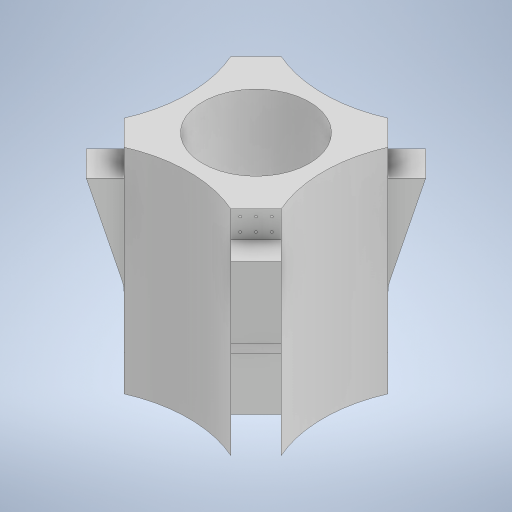
# Autodesk Inventor part: Table Base X1
Saved by Autodesk Inventor 2023 (Build 270158000, 158)
## iProperties
Created: 2022-11-22
Part Number: Table Base X1
Material: Generic
Document SubType Name: Modeling
Designer: surat
Density: 1 g/cm^3
Appearance: Default
Author: surat
Autodesk Inventor part; units mm, degrees
ref_plane "YZ Plane" through (0, 0, 0) normal (1, 0, 0) x (0, 1, 0)
ref_plane "XZ Plane" through (0, 0, 0) normal (0, 1, 0) x (-1, 0, 0)
sketch "Sketch1" plane through (0, 0, 0) normal (0, 1, 0) x (-1, 0, 0)
  line L0 (6.35, 0) -> (1365.25, 0)
  line L1 (1371.6, -6.35) -> (1371.6, -1365.25)
  line L2 (1365.25, -1371.6) -> (6.35, -1371.6)
  line L3 (0, -1365.25) -> (0, -6.35)
  line L4 (1346.2, -1346.2) -> (1346.2, -25.4)
  line L5 (1346.2, -25.4) -> (25.4, -25.4)
  line L6 (25.4, -25.4) -> (25.4, -1346.2)
  line L7 (25.4, -1346.2) -> (1346.2, -1346.2)
  line L8 (1320.8, -50.8) -> (1320.8, -1320.8)
  line L9 (1320.8, -1320.8) -> (50.8, -1320.8)
  line L10 (50.8, -1320.8) -> (50.8, -50.8)
  line L11 (50.8, -50.8) -> (1320.8, -50.8)
  line L12 (1320.8, -50.8) -> (1346.2, -25.4)
  line L13 (1320.8, -1320.8) -> (1346.2, -1346.2)
  line L14 (50.8, -1320.8) -> (25.4, -1346.2)
  line L15 (50.8, -50.8) -> (25.4, -25.4)
  line L16 (1365.25, 0) -> (1371.6, -6.35)
  line L17 (1371.6, -1365.25) -> (1365.25, -1371.6)
  line L18 (6.35, -1371.6) -> (0, -1365.25)
  line L19 (6.35, 0) -> (0, -6.35)
  line L20 (1320.8, -50.8) -> (50.8, -1320.8)
  line L21 (1320.8, -1320.8) -> (50.8, -50.8)
  line L22 (1320.8, -122.642049) -> (122.642049, -1320.8)
  line L23 (50.8, -1248.957951) -> (1248.957951, -50.8)
  line L24 (50.8, -122.642049) -> (1248.957951, -1320.8)
  line L25 (1320.8, -1248.957951) -> (122.642049, -50.8)
  line L26 (910.042049, -533.4) -> (910.042049, -838.2)
  line L27 (838.2, -910.042049) -> (533.4, -910.042049)
  line L28 (461.557951, -838.2) -> (461.557951, -533.4)
  line L29 (838.2, -461.557951) -> (533.4, -461.557951)
  line L30 (838.2, -461.557951) -> (910.042049, -533.4)
  line L31 (910.042049, -838.2) -> (838.2, -910.042049)
  line L32 (533.4, -910.042049) -> (461.557951, -838.2)
  line L33 (461.557951, -533.4) -> (533.4, -461.557951)
  arc A0 (910.042049, -533.4) -> (910.042049, -838.2) centre (1259.234317, -685.8) ccw
  arc A1 (838.2, -910.042049) -> (533.4, -910.042049) centre (685.8, -1259.234317) ccw
  arc A2 (461.557951, -838.2) -> (461.557951, -533.4) centre (112.365683, -685.8) ccw
  arc A3 (533.4, -461.557951) -> (838.2, -461.557951) centre (685.8, -112.365683) ccw
  point P0 (0, 0)
  point P1 (1371.6, -1371.6)
  point P2 (1371.6, 0)
  point P3 (0, -1371.6)
  dimension "d0" = 1371.6
  dimension "d1" = 1371.6
  dimension "d2" = 25.4
  dimension "d3" = 25.4
  dimension "d34" = 6.35
  dimension "d35" = 6.35
  dimension "d36" = 6.35
  dimension "d37" = 6.35
  dimension "d38" = 6.35
  dimension "d39" = 6.35
  dimension "d40" = 6.35
  dimension "d41" = 6.35
  dimension "d42" = 50.8
  dimension "d43" = 50.8
  dimension "d44" = 50.8
  dimension "d45" = 50.8
  dimension "d46" = 304.8
  dimension "d47" = 304.8
  dimension "d48" = 304.8
  dimension "d50" = 304.8
  dimension "d51" = 381
  dimension "d52" = 381
  dimension "d53" = 381
  dimension "d54" = 381
  constraints: 68 end point, 26 point on line, 10 parallel, 10 perpendicular, 8 point on circle, 4 centre point, 2 horizontal, 1 vertical, 6 other
  measures "d0" distance of point (1371.6, -1371.6) point (0, -1371.6)
  measures "d1" distance of point (1371.6, 0) point (1371.6, -1371.6)
  measures "d2" distance between parallel lines of L1 L4
  measures "d3" distance between parallel lines of L4 L8
  measures "d34" distance of L0.end point (1371.6, 0)
  measures "d35" distance of L1.start point (1371.6, 0)
  measures "d36" distance of L1.end point (1371.6, -1371.6)
  measures "d37" distance of L2.start point (1371.6, -1371.6)
  measures "d38" distance of L2.end point (0, -1371.6)
  measures "d39" distance of L3.start point (0, -1371.6)
  measures "d40" distance of L0.start point (0, 0)
  measures "d41" distance of L3.end point (0, 0)
  measures "d42" distance between parallel lines of L21 L25
  measures "d43" distance between parallel lines of L24 L21
  measures "d44" distance between parallel lines of L23 L20
  measures "d45" distance between parallel lines of L22 L20
  measures "d46" distance of L26.start L26.end
  measures "d47" distance of L27.start L27.end
  measures "d48" distance of L28.start L28.end
  measures "d50" distance of L29.start L29.end
  measures "d51" radius of A0
  measures "d52" radius of A1
  measures "d53" radius of A2
  measures "d54" radius of A3
sketch "Sketch2" plane through (0, 0, 0) normal (0, 1, 0) x (-1, 0, 0)
  point P0 (0, 0)
extrude "Extrusion1" add sketch "Sketch1" along normal blind 431.8 contours L31 L24 L22 L21 | L21 L22 L25 L31 | L30 L22 L25 L20 | L20 L25 L23 L30 | L32 L23 L24 L20 | L20 L24 L22 L32 | L25 L22 A0 | A1 L22 L24 | L22 L24 L20 L21 | L21 L20 L25 L22 | L33 L25 L23 L21 | L21 L23 L24 L33 | L23 L25 A3 | L20 L21 L23 L25 | A2 L24 L23 | L24 L23 L21 L20
ref_plane "Work Plane1" through (-721.721024, 0, -721.721024) normal (0.7071068, 0, -0.7071068) x (-0.7071068, 0, -0.7071068)
ref_plane "Work Plane2" through (-721.721024, 0, -649.878976) normal (-0.7071068, 0, -0.7071068) x (-0.7071068, 0, 0.7071068)
sketch "Sketch4" plane through (-721.721024, 0, -721.721024) normal (0.7071068, 0, -0.7071068) x (-0.7071068, 0, -0.7071068)
  line L0 (-317.126147, 0) -> (-317.126147, 431.8)
  line L1 (-317.126147, 431.8) -> (-317.126147, 355.6)
  line L2 (-317.126147, 355.6) -> (-555.958412, 355.6)
  line L3 (-555.958412, 355.6) -> (-563.221807, -26.378212)
  line L4 (-563.221807, -26.378212) -> (-317.126147, -18.397618)
  line L5 (-317.126147, -18.397618) -> (-387.648734, 42.02688)
  line L6 (-387.648734, 42.02688) -> (-317.126147, 101.6)
  line L7 (-317.126147, 0) -> (-101.6, 0)
  arc A0 (-317.126147, 101.6) -> (-317.126147, 355.6) centre (-424.407893, 228.6) ccw
  line L8 (0, 431.8) -> (-101.6, 431.8)
  line L9 (-50.8, 431.8) -> (-50.8, 0)
  line L10 (0, 0) -> (-101.6, 0)
  line L11 (-502.280554, 355.6) -> (-502.280554, -23.38604)
  line L12 (-502.280554, -23.38604) -> (-499.527242, -24.312672)
  point P0 (-1020.667661, 0)
  point P1 (-317.126147, 101.6)
  dimension "d64" = 76.2
  dimension "d65" = 101.6
  constraints: 18 end point, 5 point on line, 2 midpoint, 2 point on circle, 1 centre point, 1 perpendicular, 1 tangent, 1 vertical
  measures "d64" distance of L0.end L1.end
  measures "d65" distance from line of L7 L6.end
revolve "Revolution3" cut sketch "Sketch4" angle 360 about axis through (-685.8, 431.8, -685.8) along (0, -1, 0) contours L11 L12 L4 L3 L2
sketch "Sketch5" plane through (-910.042049, 355.6, -838.2) normal (-0.7071068, 0, -0.7071068) x (-0.7071068, 0, 0.7071068)
  circle A0 centre (-82.55, 57.15) radius 3.175
  circle A1 centre (-50.8, 57.15) radius 3.175
  circle A2 centre (-19.05, 57.15) radius 3.175
  circle A3 centre (-19.05, 19.05) radius 3.175
  circle A4 centre (-50.8, 19.05) radius 3.175
  circle A5 centre (-82.55, 19.05) radius 3.175
  line L0 (-50.8, 0) -> (0, 0) projected
  line L1 (-101.6, 0) -> (0, 0) projected
  line L2 (-101.6, 76.2) -> (0, 76.2) projected
  line L3 (0, -355.6) -> (0, 76.2) projected
  line L4 (-101.6, -355.6) -> (-101.6, 76.2) projected
  point P0 (-50.8, -355.6)
  dimension "d68" = 6.35
  dimension "d69" = 6.35
  dimension "d70" = 6.35
  dimension "d71" = 6.35
  dimension "d72" = 6.35
  dimension "d73" = 6.35
  dimension "d74" = 19.05
  dimension "d75" = 19.05
  dimension "d76" = 19.05
  dimension "d77" = 19.05
  dimension "d78" = 19.05
  dimension "d79" = 19.05
  dimension "d80" = 19.05
  dimension "d81" = 19.05
  dimension "d82" = 19.05
  dimension "d83" = 19.05
  dimension "d84" = 50.8
  dimension "d85" = 50.8
  constraints: 6 centre point
  measures "d68" diameter of A0
  measures "d69" diameter of A1
  measures "d70" diameter of A2
  measures "d71" diameter of A3
  measures "d72" diameter of A4
  measures "d73" diameter of A5
  measures "d74" distance from line of L0 A3.centre
  measures "d75" distance from line of L1 A4.centre
  measures "d76" distance from line of L1 A5.centre
  measures "d77" distance from line of L2 A0.centre
  measures "d78" distance from line of L2 A1.centre
  measures "d79" distance from line of L2 A2.centre
  measures "d80" distance from line of L3 A2.centre
  measures "d81" distance from line of L3 A3.centre
  measures "d82" distance from line of L4 A5.centre
  measures "d83" distance from line of L4 A0.centre
  measures "d84" distance from line of L4 A1.centre
  measures "d85" distance from line of L4 A4.centre
extrude "Extrusion2" cut sketch "Sketch5" against normal blind 50.8 contours A0 | A1 | A2 | A3 | A4 | A5
pattern_circular "Circular Pattern1" count 4 over 360 about axis through (-685.8, 0, -685.8) along (0, 1, 0) of "Extrusion2"
ref_plane "Work Plane3" through (0, 355.6, 0) normal (0, 1, 0) x (1, 0, 0)
sketch "Sketch6" plane through (0, 355.6, 0) normal (0, 1, 0) x (1, 0, 0)
  line L0 (-533.4, 461.557951) -> (-461.557951, 533.4)
  line L1 (-461.557951, 533.4) -> (-407.676414, 479.518463)
  arc A0 (-533.4, 461.557951) -> (-838.2, 461.557951) centre (-685.8, 112.365683) ccw
  line L2 (-533.4, 461.557951) -> (-479.518463, 407.676414)
  line L3 (-407.676414, 479.518463) -> (-479.518463, 407.676414)
  line L4 (-461.557951, 533.4) -> (-533.4, 461.557951)
  point P0 (0, 0)
  dimension "d92" = 76.2
  dimension "d93" = 76.2
  constraints: 8 end point, 2 perpendicular
  measures "d92" distance of L0.end L1.end
  measures "d93" distance of L0.start L2.end
sketch "Sketch7" plane through (-461.557951, 0, -533.4) normal (0.7071068, 0, 0.7071068) x (0.7071068, 0, -0.7071068)
  line L0 (0, 0) -> (0, 431.8)
  line L1 (-101.6, 355.558582) -> (0, 355.558582)
  line L2 (0, 355.558582) -> (0, 88.9)
  line L3 (0, 88.9) -> (-101.6, 88.9)
  line L4 (-101.6, 88.9) -> (-101.6, 355.558582)
  line L5 (-101.6, 0) -> (0, 0)
  point P0 (-50.8, 0)
  dimension "d94" = 88.9
  constraints: 8 end point, 2 parallel, 1 horizontal, 1 perpendicular, 1 point on line
  measures "d94" distance between parallel lines of L3 L5
loft "Loft1" add profiles "Sketch6", "Sketch7"
pattern_circular "Circular Pattern2" count 4 over 360 about axis through (-685.8, 0, -685.8) along (0, 1, 0) of "Loft1"
fillet "Fillet2" radius 101.6 4 edges at (-874.121, 88.9, -497.479) (-497.479, 88.9, -497.479) (-497.479, 88.9, -874.121) (-874.121, 88.9, -874.121)
sketch "Sketch8" plane through (0, 0, 0) normal (0, -1, 0) x (1, 0, 0)
  arc A0 (-461.557951, -533.4) -> (-461.557951, -838.2) centre (-112.365683, -685.8) ccw
  line L0 (-838.2, -461.557951) -> (-461.557951, -838.2)
  line L1 (-838.2, -910.042049) -> (-892.081537, -963.923586)
  line L2 (-461.557951, -533.4) -> (-838.2, -910.042049)
  line L3 (-533.4, -461.557951) -> (-461.557951, -533.4)
  line L4 (-533.4, -461.557951) -> (-461.557951, -533.4)
  arc A1 (-533.4, -910.042049) -> (-838.2, -910.042049) centre (-685.8, -1259.234317) ccw
  arc A2 (-838.2, -461.557951) -> (-533.4, -461.557951) centre (-685.8, -112.365683) ccw
  line L5 (-910.042049, -533.4) -> (-838.2, -461.557951)
  arc A3 (-910.042049, -838.2) -> (-910.042049, -533.4) centre (-1259.234317, -685.8) ccw
  line L6 (-838.2, -910.042049) -> (-910.042049, -838.2)
  arc A4 (-533.4, -910.042049) -> (-838.2, -910.042049) centre (-685.8, -1259.234317) ccw
  line L7 (-461.557951, -838.2) -> (-533.4, -910.042049)
  arc A5 (-461.557951, -533.4) -> (-461.557951, -838.2) centre (-112.365683, -685.8) ccw
  line L8 (-533.4, -461.557951) -> (-461.557951, -533.4)
  line L9 (-910.042049, -533.4) -> (-838.2, -461.557951)
  line L10 (-910.042049, -533.4) -> (-533.4, -910.042049)
  line L11 (-522.17468, -898.816729) -> (-558.095704, -862.895704)
  line L12 (-910.042049, -838.2) -> (-533.4, -461.557951)
  point P0 (0, 0)
  point P1 (-458.793753, -840.964198)
  point P2 (-533.4, -910.042049)
  point P3 (-685.8, -757.642049)
  point P4 (-613.957951, -685.8)
  point P5 (-757.642049, -685.8)
  point P6 (-533.4, -461.557951)
  point P7 (-685.8, -613.957951)
  constraints: 10 end point, 2 collinear, 1 parallel, 1 perpendicular
extrude "Extrusion3" add sketch "Sketch8" along normal blind 177.8 contours A0 L0 L2 | L12 L0 A2 | L10 A1 L2 | L12 A3 L10
sketch "Sketch9" plane through (0, 0, 0) normal (0, -1, 0) x (1, 0, 0)
  line L0 (-461.557951, -838.2) -> (-613.957951, -685.8)
  line L1 (-613.957951, -685.8) -> (-461.557951, -533.4)
  line L2 (-533.4, -461.557951) -> (-461.557951, -533.4)
  line L3 (-533.4, -461.557951) -> (-685.8, -613.957951)
  line L4 (-685.8, -613.957951) -> (-838.2, -461.557951)
  line L5 (-910.042049, -533.4) -> (-838.2, -461.557951)
  line L6 (-910.042049, -533.4) -> (-757.642049, -685.8)
  line L7 (-757.642049, -685.8) -> (-910.042049, -838.2)
  line L8 (-838.2, -910.042049) -> (-910.042049, -838.2)
  line L9 (-838.2, -910.042049) -> (-685.8, -757.642049)
  line L10 (-685.8, -757.642049) -> (-533.4, -910.042049)
  line L11 (-461.557951, -838.2) -> (-533.4, -910.042049)
  point P0 (0, 0)
extrude "Extrusion4" add sketch "Sketch9" along normal blind 76.2
sketch "Sketch10" plane through (0, -76.2, 0) normal (0, -1, 0) x (1, 0, 0)
  line L0 (-894.326601, -853.915448) -> (-858.405576, -817.994424)
  circle A0 centre (-876.366089, -835.954936) radius 3.175
  circle A1 centre (-838.2, -874.121024) radius 3.175
  circle A2 centre (-802.278976, -838.2) radius 3.175
  circle A3 centre (-838.2, -802.278976) radius 3.175
  circle A4 centre (-838.2, -838.2) radius 3.175
  line L1 (-910.042049, -838.2) -> (-838.2, -910.042049)
  line L2 (-685.8, -757.642049) -> (-838.2, -910.042049)
  line L3 (-910.042049, -838.2) -> (-757.642049, -685.8)
  point P0 (0, 0)
  dimension "d107" = 6.35
  dimension "d109" = 6.35
  dimension "d110" = 6.35
  dimension "d112" = 6.35
  dimension "d113" = 6.35
  dimension "d114" = 25.4
  dimension "d115" = 25.4
  dimension "d116" = 25.4
  dimension "d117" = 76.2
  dimension "d118" = 76.2
  dimension "d119" = 25.4
  dimension "d120" = 25.4
  dimension "d121" = 50.8
  dimension "d122" = 50.8
  constraints: 5 centre point, 1 midpoint
  measures "d107" diameter of A0
  measures "d109" diameter of A1
  measures "d110" diameter of A2
  measures "d112" diameter of A3
  measures "d113" diameter of A4
  measures "d114" distance from line of L1 A1.centre
  measures "d115" distance from line of L2 A1.centre
  measures "d116" distance from line of L2 A2.centre
  measures "d117" distance from line of L1 A2.centre
  measures "d118" distance from line of L1 A3.centre
  measures "d119" distance from line of L3 A3.centre
  measures "d120" distance from line of L1 A0.centre
  measures "d121" distance from line of L1 A4.centre
  measures "d122" distance from line of L3 A4.centre
extrude "Extrusion5" cut sketch "Sketch10" against normal blind 76.2
pattern_circular "Circular Pattern3" count 4 over 360 about axis through (-685.8, 0, -685.8) along (0, 1, 0) of "Extrusion5"
sketch "Sketch11" plane through (0, 431.8, 0) normal (0, 1, 0) x (1, 0, 0)
  circle A0 centre (-685.807853, 685.8) radius 152.4
  line L0 (-461.557951, 838.2) -> (-533.4, 910.042049)
  line L1 (-533.4, 461.557951) -> (-461.557951, 533.4)
  point P0 (0, 0)
  dimension "d128" = 304.8
  dimension "d129" = 266.3317
  dimension "d130" = 266.3317
  constraints: 1 centre point
  measures "d128" diameter of A0
  measures "d129" distance from line of L0 A0.centre
  measures "d130" distance from line of L1 A0.centre
extrude "Extrusion6" cut sketch "Sketch11" against normal blind 2032
equation "\"d35\" = d34"
equation "\"d36\" = d34"
equation "\"d37\" = d36"
equation "\"d38\" = d34"
equation "\"d39\" = d38"
equation "\"d40\" = d34"
equation "\"d41\" = d40"
body "Solid1"
